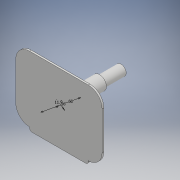
# Autodesk Inventor part: Part7
Saved by Autodesk Inventor 2018 (Build 220112000, 112)
## iProperties
Created: 2018-09-20
Part Number: Part7
Material: Generic
Document SubType Name: Modeling
Designer: ryanc
Density: 1 g/cm^3
Appearance: Default
Author: ryanc
Autodesk Inventor part; units mm, degrees
ref_plane "YZ Plane" through (0, 0, 0) normal (1, 0, 0) x (0, 1, 0)
ref_plane "XZ Plane" through (0, 0, 0) normal (0, 1, 0) x (-1, 0, 0)
ref_plane "XY Plane" through (0, 0, 0) normal (0, 0, 1) x (1, 0, 0)
sketch "Sketch1" plane through (0, 0, 0) normal (0, 1, 0) x (-1, 0, 0)
  circle A0 centre (0, 0) radius 5.95
  circle A1 centre (0, 0) radius 8
  circle A2 centre (0, 0) radius 30
  dimension "d0" = 11.9
  dimension "d2" = 16
  dimension "d3" = 60
  constraints: 5 coincident, 3 centre point
  measures "d0" diameter of A0
  measures "d2" diameter of A1
  measures "d3" diameter of A2
extrude "Extrusion1" add sketch "Sketch1" along normal blind 70 contours A0
extrude "Extrusion2" cut sketch "Sketch1" along normal blind 45 contours A1
extrude "Extrusion3" add sketch "Sketch1" along normal blind 45 contours A0 | A1
extrude "Extrusion4" add sketch "Sketch1" along normal blind 12 contours A2
sketch "Sketch2" plane through (0, 0, 0) normal (0, -1, 0) x (1, 0, 0)
  line L0 (-50, 38) -> (50, 38)
  line L1 (50, 38) -> (50, -38)
  line L2 (50, -38) -> (-50, -38)
  line L3 (-50, -38) -> (-50, 38)
  line L4 (-50, 38) -> (50, -38) construction
  line L5 (50, 38) -> (-50, -38) construction
  point P0 (0, 0)
  dimension "d12" = 100
  constraints: 12 end point, 2 midpoint, 2 parallel, 1 horizontal, 1 perpendicular
  measures "d12" distance of L1.end L2.end
extrude "Extrusion5" add sketch "Sketch2" along normal blind 2
fillet "Fillet1" radius 16 4 edges at (50, -1, 38) (50, -1, -38) (-50, -1, -38) (-50, -1, 38)
fillet "Fillet2" radius 16 1 edges at (30, 12, 0)
sketch "Sketch3" plane through (34, 0, -38) normal (0, 0, -1) x (-1, 0, 0)
  line L0 (0, 0) -> (68, 0) projected
  line L1 (0, -2) -> (68, -2)
  line L2 (68, -2) -> (68, 0)
  line L3 (68, 0) -> (0, 0)
  line L4 (0, 0) -> (0, -2)
  point P0 (34, 0)
  constraints: 8 end point, 2 parallel, 1 horizontal, 1 perpendicular
extrude "Extrusion6" add sketch "Sketch3" along normal blind 4
sketch "Sketch4" plane through (0, 0, 0) normal (0, 1, 0) x (1, 0, 0)
  line L0 (-34, 42) -> (34, 42) projected
  line L1 (-34, 38) -> (-34, 42) projected
  line L2 (34, 42) -> (-34, 42)
  line L3 (-34, 42) -> (-34, 38)
  line L4 (-34, 38) -> (34, 38)
  line L5 (34, 38) -> (34, 42)
  point P0 (0, 0)
  constraints: 8 end point, 2 parallel, 1 horizontal, 1 perpendicular
extrude "Extrusion7" add sketch "Sketch4" along normal blind 5
fillet "Fillet3" radius 3 3 edges at (0, 5, -42) (-34, 1.5, -42) (34, 1.5, -42)
fillet "Fillet4" radius 1 1 edges at (0, 5, -38)
body "Solid1"
